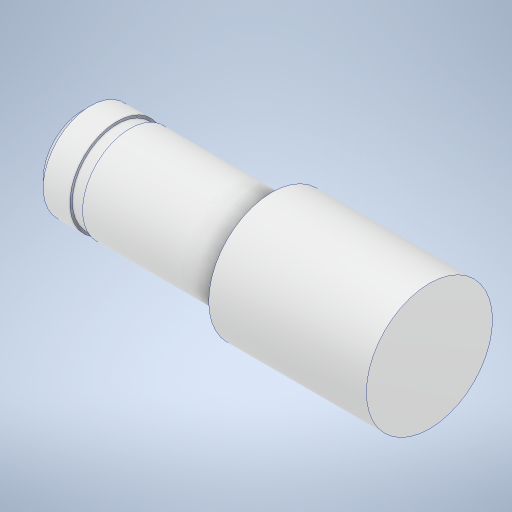
# Autodesk Inventor part: Bolt_Acht_Durchmesser
Saved by Autodesk Inventor 2024 (Build 280153000, 153)
## iProperties
Created: 2024-03-08
Part Number: Bolt_Acht_Durchmesser
Material: Aluminium 6061
Document SubType Name: Modeling
Designer: ffogue
Density: 2.7 g/cm^3
Appearance: Aluminium - flach
Author: ffogue
Autodesk Inventor part; units mm, degrees
ref_plane "YZ Plane" through (0, 0, 0) normal (1, 0, 0) x (0, 1, 0)
ref_plane "XZ Plane" through (0, 0, 0) normal (0, 1, 0) x (-1, 0, 0)
ref_plane "XY Plane" through (0, 0, 0) normal (0, 0, 1) x (1, 0, 0)
sketch "Skizze1" plane through (0, 0, 0) normal (0, 0, 1) x (1, 0, 0)
  line L0 (0, 0) -> (22, 0)
  line L1 (0, 0) -> (0, 3)
  line L2 (0, 3) -> (2.2, 3)
  line L3 (2.2, 3) -> (2.2, 2.85)
  line L4 (2.2, 2.85) -> (3, 2.85)
  line L5 (3, 2.85) -> (3, 3)
  line L6 (3, 3) -> (12, 3)
  line L7 (12, 3) -> (12, 4)
  line L8 (12, 4) -> (22, 4)
  line L9 (22, 4) -> (22, 0)
  dimension "d0" = 22
  dimension "d1" = 10
  dimension "d2" = 9
  dimension "d3" = 0.8
  dimension "d4" = 8
  dimension "d5" = 6
  dimension "d6" = 5.7
  constraints: 20 end point, 7 perpendicular, 2 point on line, 1 coincident, 1 horizontal, 1 vertical
  measures "d0" distance of L0.start L0.end
  measures "d1" distance between parallel lines of L9 L7
  measures "d2" distance between parallel lines of L7 L5
  measures "d3" distance between parallel lines of L5 L3
  measures "d4" diameter of L8.end L0
  measures "d5" diameter of L6 L0
  measures "d6" diameter of L4 L0
revolve "Umdrehung1" add sketch "Skizze1" angle 360 about axis through (0, 0, 0) along (1, 0, 0)
chamfer "Fasen1" distance 0.5 angle 45 1 edges at (0, -3, 0)
